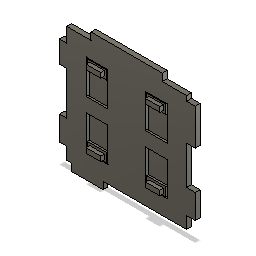
LCD_spring_holder (Autodesk Fusion 360 design; units mm, degrees)
Autodesk Fusion 360 part; units mm, degrees
sketch "Sketch1" plane through (0, 0, 0) normal (0, 0, 1) x (1, 0, 0)
  line L0 (0, 47.8) -> (49.4, 47.8)
  line L1 (49.4, 47.8) -> (49.4, 0)
  line L2 (49.4, 0) -> (0, 0)
  line L3 (0, 0) -> (0, 47.8)
  line L4 (10, 47.8) -> (10, 50.8)
  line L5 (10, 50.8) -> (39.4, 50.8)
  line L6 (39.4, 50.8) -> (39.4, 47.8)
  line L7 (49.4, 45.8) -> (53, 45.8)
  line L8 (53, 45.8) -> (53, 30.8)
  line L9 (53, 30.8) -> (49.4, 30.8)
  line L10 (49.4, 15) -> (53, 15)
  line L11 (53, 15) -> (53, 5)
  line L12 (53, 5) -> (49.4, 5)
  line L13 (0, 41.8) -> (-3, 41.8)
  line L14 (-3, 41.8) -> (-3, 32.8)
  line L15 (-3, 32.8) -> (0, 32.8)
  line L16 (2, 0) -> (2, -3)
  line L17 (2, -3) -> (15, -3)
  line L18 (15, -3) -> (15, 0)
  line L19 (0, 5) -> (-3, 5)
  line L20 (-3, 5) -> (-3, 15)
  line L21 (-3, 15) -> (0, 15)
  line L22 (8.5, 36.8) -> (8.5, 26.8)
  line L23 (8.5, 26.8) -> (8, 26.8)
  line L24 (8, 26.8) -> (8, 40.8)
  line L25 (8, 40.8) -> (17, 40.8)
  line L26 (17, 40.8) -> (17, 26.8)
  line L27 (17, 26.8) -> (16.5, 26.8)
  line L28 (16.5, 26.8) -> (16.5, 36.8)
  line L29 (16.5, 36.8) -> (8.5, 36.8)
  line L30 (9.5, 39.8) -> (9.5, 37.8)
  line L31 (9.5, 37.8) -> (15.5, 37.8)
  line L32 (15.5, 37.8) -> (15.5, 39.8)
  line L33 (15.5, 39.8) -> (9.5, 39.8)
  line L34 (8.5, 36.8) -> (8.5, 40.4566)
  line L35 (8.5, 40.4566) -> (16.5, 40.4566)
  line L36 (16.5, 40.4566) -> (16.5, 36.8)
  line L37 (8.5, 26.8) -> (16.5, 26.8)
  line L38 (33.9, 39.8) -> (33.9, 37.8)
  line L39 (32.9, 36.8) -> (32.9, 40.4566)
  line L40 (32.9, 26.8) -> (32.4, 26.8)
  line L41 (32.4, 26.8) -> (32.4, 40.8)
  line L42 (40.9, 26.8) -> (40.9, 36.8)
  line L43 (40.9, 36.8) -> (32.9, 36.8)
  line L44 (32.4, 40.8) -> (41.4, 40.8)
  line L45 (40.9, 40.4566) -> (40.9, 36.8)
  line L46 (32.9, 36.8) -> (32.9, 26.8)
  line L47 (41.4, 40.8) -> (41.4, 26.8)
  line L48 (32.9, 40.4566) -> (40.9, 40.4566)
  line L49 (41.4, 26.8) -> (40.9, 26.8)
  line L50 (32.9, 26.8) -> (40.9, 26.8)
  line L51 (33.9, 37.8) -> (39.9, 37.8)
  line L52 (39.9, 37.8) -> (39.9, 39.8)
  line L53 (39.9, 39.8) -> (33.9, 39.8)
  line L54 (16.5, 11) -> (16.5, 7.3434)
  line L55 (40.9, 11) -> (40.9, 7.3434)
  line L56 (39.9, 8) -> (39.9, 10)
  line L57 (16.5, 21) -> (17, 21)
  line L58 (41.4, 21) -> (41.4, 7)
  line L59 (15.5, 10) -> (9.5, 10)
  line L60 (32.9, 11) -> (40.9, 11)
  line L61 (16.5, 11) -> (16.5, 21)
  line L62 (15.5, 8) -> (15.5, 10)
  line L63 (40.9, 21) -> (41.4, 21)
  line L64 (9.5, 8) -> (15.5, 8)
  line L65 (40.9, 11) -> (40.9, 21)
  line L66 (16.5, 7.3434) -> (8.5, 7.3434)
  line L67 (40.9, 21) -> (32.9, 21)
  line L68 (32.4, 21) -> (32.9, 21)
  line L69 (9.5, 10) -> (9.5, 8)
  line L70 (41.4, 7) -> (32.4, 7)
  line L71 (33.9, 8) -> (39.9, 8)
  line L72 (40.9, 7.3434) -> (32.9, 7.3434)
  line L73 (39.9, 10) -> (33.9, 10)
  line L74 (32.9, 7.3434) -> (32.9, 11)
  line L75 (33.9, 10) -> (33.9, 8)
  line L76 (17, 21) -> (17, 7)
  line L77 (8, 7) -> (8, 21)
  line L78 (32.4, 7) -> (32.4, 21)
  line L79 (8.5, 7.3434) -> (8.5, 11)
  line L80 (16.5, 21) -> (8.5, 21)
  line L81 (8.5, 21) -> (8.5, 11)
  line L82 (17, 7) -> (8, 7)
  line L83 (32.9, 21) -> (32.9, 11)
  line L84 (8, 21) -> (8.5, 21)
  line L85 (8.5, 11) -> (16.5, 11)
  point P0 (24.7, 23.9)
  dimension "d1" = 49.4
  dimension "d2" = 47.8
  dimension "d3" = 2
  dimension "d4" = 15
  dimension "d5" = 3
  dimension "d6" = 5
  dimension "d7" = 10
  dimension "d8" = 3
  dimension "d9" = 6
  dimension "d10" = 15
  dimension "d11" = 3
  dimension "d12" = 10
  dimension "d13" = 10
  dimension "d14" = 3
  dimension "d15" = 2
  dimension "d16" = 15
  dimension "d17" = 5
  dimension "d18" = 10
  dimension "d19" = 0.5
  dimension "d20" = 0.5
  dimension "d21" = 10
  dimension "d23" = 1
  dimension "d24" = 1
  dimension "d26" = 2
  dimension "d27" = 1
  dimension "d28" = 1
  dimension "d29" = 7
  dimension "d30" = 8
  dimension "d31" = 24.7
  dimension "d32" = 23.9
  dimension "d33" = 8
  dimension "d34" = 9
  dimension "d37" = 24.4
  dimension "d38" = 0
  dimension "d40" = 360
  constraint horizontal L0
  constraint perpendicular L0 L1
  constraint coincident L2.end L3.start
  constraint perpendicular L1 L2
  constraint perpendicular L0 L3
  constraint coincident L0 L4.start
  constraint perpendicular L0 L4
  constraint perpendicular L4 L5
  constraint coincident L0 L6.end
  constraint perpendicular L0 L6
  constraint coincident L1 L7.start
  constraint perpendicular L1 L7
  constraint perpendicular L7 L8
  constraint coincident L1 L9.end
  constraint perpendicular L8 L9
  constraint coincident L1 L10.start
  constraint perpendicular L1 L10
  constraint perpendicular L7 L11
  constraint coincident L1 L12.end
  constraint perpendicular L1 L12
  constraint coincident L3 L13.start
  constraint perpendicular L3 L13
  constraint perpendicular L13 L14
  constraint coincident L3 L15.end
  constraint perpendicular L3 L15
  constraint coincident L2 L16.start
  constraint perpendicular L2 L16
  constraint perpendicular L3 L17
  constraint coincident L2 L18.end
  constraint perpendicular L2 L18
  constraint coincident L3 L19.start
  constraint perpendicular L3 L19
  constraint perpendicular L19 L20
  constraint coincident L3 L21.end
  constraint perpendicular L3 L21
  constraint vertical L22
  constraint perpendicular L22 L23
  constraint perpendicular L23 L24
  constraint perpendicular L24 L25
  constraint perpendicular L25 L26
  constraint perpendicular L24 L27
  constraint perpendicular L27 L28
  constraint perpendicular L28 L29
  constraint equal L22 L28
  constraint vertical L30
  constraint perpendicular L30 L31
  constraint perpendicular L31 L32
  constraint perpendicular L32 L33
  constraint perpendicular L29 L34
  constraint perpendicular L34 L35
  constraint perpendicular L29 L36
  measures "d1" distance of L1 L3
  measures "d2" distance of L0 L2
  measures "d3" distance of L3 L16
  measures "d4" distance of L3 L18
  measures "d5" distance of L2 L17
  measures "d6" distance of L2 L19
  measures "d7" distance of L19 L21
  measures "d8" distance of L3 L20
  measures "d9" distance of L0 L13
  measures "d10" distance of L0 L15
  measures "d11" distance of L3 L14
  measures "d12" distance of L3 L4
  measures "d13" distance of L1 L6
  measures "d14" distance of L0 L5
  measures "d15" distance of L0 L7
  measures "d16" distance of L7 L9
  measures "d17" distance of L2 L12
  measures "d18" distance of L10 L12
  measures "d19" distance of L26 L28
  measures "d20" distance of L22 L24
  measures "d21" distance of L27 L29
  measures "d23" distance of L25 L33
  measures "d24" distance of L29 L31
  measures "d26" distance of L31 L33
  measures "d27" distance of L30 L34
  measures "d28" distance of L32 L36
  measures "d29" distance of L0 L25
  measures "d30" distance of L3 L24
  measures "d31" distance of L3 P0
  measures "d32" distance of L2 P0
  measures "d33" distance of L22 L28
  measures "d34" distance of L24 L26
extrude "Extrude1" add sketch "Sketch1" along normal blind 2 contours L0 L1 L2 L3 | L0 L4 L5 L6 | L3 L13 L14 L15 | L3 L19 L20 L21 | L1 L7 L8 L9 | L1 L10 L11 L12 | L2 L16 L17 L18 | L22 L28 L29 L37 | L29 L34 L35 L36 | L30 L31 L32 L33 | L38 L51 L52 L53 | L39 L43 L45 L48 | L42 L43 L46 L50 | L61 L80 L81 L85 | L54 L66 L79 L85 | L55 L60 L72 L74 | L60 L65 L67 L83 | L56 L71 L73 L75 | L59 L62 L64 L69
extrude "Extrude2" cut sketch "Sketch1" against normal blind 0.8 from surface at 2 contours L22 L28 L29 L37 | L42 L43 L46 L50 | L61 L80 L81 L85 | L60 L65 L67 L83
extrude "Extrude3" add sketch "Sketch1" along normal blind 1.5 from surface at 2 contours L30 L31 L32 L33 | L38 L51 L52 L53 | L56 L71 L73 L75 | L59 L62 L64 L69
